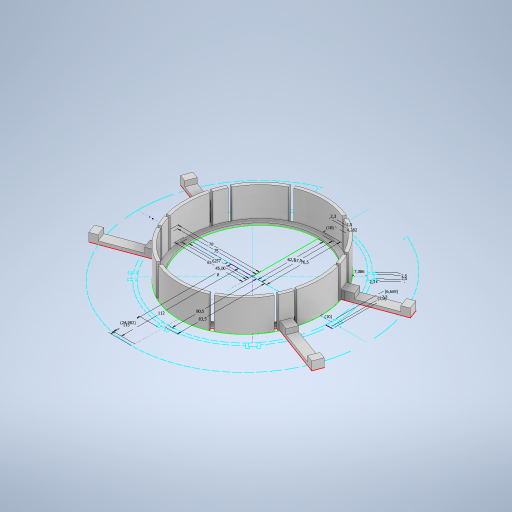
# Autodesk Inventor part: calibracao(0,5cm)
Saved by Autodesk Inventor 2024.3 (Build 283343000, 343)
## iProperties
Created: 2024-12-11
Part Number: calibracao(0,5cm)
Material: Genérico
Document SubType Name: Modeling
Designer: lostv
Density: 1 g/cm^3
Appearance: Padrão
Author: lostv
Autodesk Inventor part; units mm, degrees
ref_plane "YZ Plane" through (0, 0, 0) normal (1, 0, 0) x (0, 1, 0)
ref_plane "XZ Plane" through (0, 0, 0) normal (0, 1, 0) x (-1, 0, 0)
ref_plane "XY Plane" through (0, 0, 0) normal (0, 0, 1) x (1, 0, 0)
sketch "Esboço1" plane through (0, 0, 0) normal (0, 1, 0) x (-1, 0, 0)
  ellipse E0 centre (-16.8231, 43.9447) end of major axis (58.1769, 43.9447) minor radius 80.5 (58.1769, 43.9447) -> (-16.8231, 124.4447) ccw
  line L0 (-16.8231, 124.4447) -> (-16.8231, 43.9447) construction
  line L1 (-16.8231, 43.9447) -> (58.1769, 43.9447)
  line L2 (-16.8231, 43.9447) -> (38.0514, 98.8191) construction
  line L3 (-16.8231, 43.9447) -> (60.7811, 43.9447) construction
  line L4 (58.1769, 43.9447) -> (61.1769, 43.9447)
  ellipse E1 centre (-16.8231, 43.9447) end of major axis (-16.8231, 127.4447) minor radius 78 (36.942, 104.4388) -> (-11.8231, 127.273) ccw
  ellipse E2 centre (-16.8231, 43.9447) end of major axis (-16.8231, 127.4447) minor radius 78 (61.0369, 48.9447) -> (43.4965, 96.8842) ccw
  ellipse E3 centre (-16.8231, 43.9447) end of major axis (-16.8231, 127.4447) minor radius 78 (-21.8231, 127.273) -> (-70.5882, 104.4388) ccw
  ellipse E4 centre (-16.8231, 43.9447) end of major axis (-91.8231, 43.9447) minor radius 80.5 (-16.8231, 124.4447) -> (-91.8231, 43.9447) ccw
  line L5 (-16.8231, 43.9447) -> (-71.6976, 98.8191) construction
  line L6 (-16.8231, 43.9447) -> (-91.8231, 43.9447) construction
  line L7 (-16.8231, 43.9447) -> (-91.8231, 43.9447)
  ellipse E5 centre (-16.8231, 43.9447) end of major axis (-16.8231, 127.4447) minor radius 78 (-77.1427, 96.8842) -> (-94.6831, 48.9447) ccw
  line L8 (-96.047, 46.9447) -> (-91.771, 46.9447)
  line L9 (58.1769, 43.9447) -> (-91.8231, 43.9447)
  line L10 (-16.8231, 43.9447) -> (38.0514, -10.9298) construction
  ellipse E6 centre (-16.8231, 43.9447) end of major axis (58.1769, 43.9447) minor radius 80.5 (-16.8231, -36.5553) -> (58.1769, 43.9447) ccw
  line L11 (-16.8231, -36.5553) -> (-16.8231, 43.9447) construction
  line L12 (-13.8231, -40.7731) -> (-13.8231, -36.4909)
  line L13 (-11.8231, -40.7731) -> (-11.8231, -36.3762)
  line L14 (-13.8231, -36.4909) -> (-13.8231, -40.7731)
  ellipse E7 centre (-16.8231, 43.9447) end of major axis (-16.8231, -39.5553) minor radius 78 (-11.8231, -39.3836) -> (36.942, -16.5494) ccw
  ellipse E8 centre (-16.8231, 43.9447) end of major axis (-16.8231, -39.5553) minor radius 78 (43.4965, -8.9948) -> (61.0369, 38.9447) ccw
  line L15 (-69.7437, -13.0978) -> (-72.9021, -15.9416)
  line L16 (-73.673, -8.5619) -> (-76.9169, -11.4827)
  line L17 (-73.673, -8.5619) -> (-76.9169, -11.4827)
  line L18 (-69.7437, -13.0978) -> (-72.9021, -15.9416)
  line L19 (-19.8231, -40.7731) -> (-19.8231, -36.4909)
  line L20 (-19.8231, -36.4909) -> (-19.8231, -40.7731)
  line L21 (-21.8231, -40.7731) -> (-21.8231, -36.3762)
  ellipse E9 centre (-16.8231, 43.9447) end of major axis (-16.8231, -39.5553) minor radius 78 (-70.5882, -16.5494) -> (-21.8231, -39.3836) ccw
  line L22 (-16.8231, 43.9447) -> (-71.6976, -10.9298) construction
  ellipse E10 centre (-16.8231, 43.9447) end of major axis (-91.8231, 43.9447) minor radius 80.5 (-91.8231, 43.9447) -> (-16.8231, -36.5553) ccw
  ellipse E11 centre (-16.8231, 43.9447) end of major axis (-16.8231, -39.5553) minor radius 78 (-94.6831, 38.9447) -> (-77.1427, -8.9948) ccw
  line L23 (-96.047, 40.9447) -> (-91.8, 40.9447)
  line L24 (-56.8231, -78.0731) -> (-56.8231, -78.0731)
  line L25 (-96.047, 38.9447) -> (-91.6783, 38.9447)
  line L26 (-96.047, 48.9447) -> (-91.6783, 48.9447)
  line L27 (-96.047, 38.9447) -> (-98.347, 38.9447) construction
  line L28 (-98.347, 38.9447) -> (-98.347, 41.4447) construction
  line L29 (-98.347, 41.4447) -> (-96.047, 41.4447) construction
  line L30 (-96.047, 38.9447) -> (-98.347, 38.9447)
  line L31 (-98.347, 41.4447) -> (-98.347, 38.9447)
  line L32 (-98.347, 41.4447) -> (-96.047, 41.4447)
  line L33 (-96.047, 41.4447) -> (-96.047, 40.9447)
  line L34 (-96.047, 46.9447) -> (-96.047, 46.4447)
  line L35 (-98.347, 46.4447) -> (-96.047, 46.4447)
  line L36 (-98.347, 46.4447) -> (-98.347, 48.9447)
  line L37 (-98.347, 48.9447) -> (-96.047, 48.9447)
  line L38 (-96.047, 40.9447) -> (-96.047, 41.4447) construction
  line L39 (-96.047, 46.4447) -> (-96.047, 46.9447) construction
  line L40 (-96.047, 41.4447) -> (-96.047, 46.4447)
  line L41 (-72.9021, -15.9416) -> (-76.9169, -11.4827) construction
  line L42 (-78.2551, -9.9964) -> (-74.9072, -6.9819)
  line L43 (-71.5638, -17.4279) -> (-68.3579, -14.5413)
  line L44 (-71.5638, -17.4279) -> (-73.2731, -18.9669)
  line L45 (-73.2731, -18.9669) -> (-74.9459, -17.109)
  line L46 (-74.9459, -17.109) -> (-73.2367, -15.57)
  line L47 (-72.9021, -15.9416) -> (-73.2367, -15.57)
  line L48 (-76.9169, -11.4827) -> (-73.2367, -15.57)
  line L49 (-78.2551, -9.9964) -> (-79.9644, -11.5354)
  line L50 (-79.9644, -11.5354) -> (-78.2915, -13.3933)
  line L51 (-78.2915, -13.3933) -> (-76.5823, -11.8543)
  line L52 (-13.8231, -40.7731) -> (-19.8231, -40.7731) construction
  line L53 (-21.8231, -40.7731) -> (-21.8231, -43.0731)
  line L54 (-21.8231, -43.0731) -> (-19.3231, -43.0731)
  line L55 (-19.3231, -43.0731) -> (-19.3231, -40.7731)
  line L56 (-19.8231, -40.7731) -> (-19.3231, -40.7731)
  line L57 (-11.8231, -40.7731) -> (-11.8231, -43.0731)
  line L58 (-11.8231, -43.0731) -> (-14.3231, -43.0731)
  line L59 (-14.3231, -43.0731) -> (-14.3231, -40.7731)
  line L60 (-13.8231, -40.7731) -> (-14.3231, -40.7731)
  line L61 (-19.3231, -40.7731) -> (-14.3231, -40.7731)
  line L62 (46.3182, -11.5354) -> (44.6453, -13.3933)
  line L63 (44.6089, -9.9964) -> (46.3182, -11.5354)
  line L64 (44.6453, -13.3933) -> (42.9361, -11.8543)
  line L65 (40.0268, -8.5619) -> (43.2707, -11.4827)
  line L66 (44.6089, -9.9964) -> (41.261, -6.9819)
  line L67 (43.2707, -11.4827) -> (39.5905, -15.57)
  line L68 (39.2559, -15.9416) -> (43.2707, -11.4827) construction
  line L69 (36.0975, -13.0978) -> (39.2559, -15.9416)
  line L70 (39.2559, -15.9416) -> (39.5905, -15.57)
  line L71 (41.2997, -17.109) -> (39.5905, -15.57)
  line L72 (39.6269, -18.9669) -> (41.2997, -17.109)
  line L73 (37.9176, -17.4279) -> (39.6269, -18.9669)
  line L74 (37.9176, -17.4279) -> (34.7117, -14.5413)
  line L75 (62.4009, 38.9447) -> (64.7009, 38.9447)
  line L76 (64.7009, 38.9447) -> (64.7009, 41.4447)
  line L77 (64.7009, 41.4447) -> (62.4009, 41.4447)
  line L78 (62.4009, 41.4447) -> (62.4009, 40.9447)
  line L79 (62.4009, 40.9447) -> (58.1538, 40.9447)
  line L80 (62.4009, 38.9447) -> (58.0321, 38.9447)
  line L81 (62.4009, 41.4447) -> (62.4009, 46.4447)
  line L82 (64.7009, 46.4447) -> (62.4009, 46.4447)
  line L83 (62.4009, 46.9447) -> (62.4009, 46.4447)
  line L84 (64.7009, 46.4447) -> (64.7009, 48.9447)
  line L85 (64.7009, 48.9447) -> (62.4009, 48.9447)
  line L86 (62.4009, 48.9447) -> (58.0321, 48.9447)
  line L87 (62.4009, 46.9447) -> (58.1248, 46.9447)
  line L88 (39.2559, 103.831) -> (39.5905, 103.4594)
  line L89 (37.9176, 105.3172) -> (39.6269, 106.8562)
  line L90 (39.6269, 106.8562) -> (41.2997, 104.9984)
  line L91 (41.2997, 104.9984) -> (39.5905, 103.4594)
  line L92 (39.2559, 103.831) -> (43.2707, 99.3721) construction
  line L93 (43.2707, 99.3721) -> (39.5905, 103.4594)
  line L94 (44.6453, 101.2827) -> (42.9361, 99.7437)
  line L95 (46.3182, 99.4248) -> (44.6453, 101.2827)
  line L96 (44.6089, 97.8858) -> (46.3182, 99.4248)
  line L97 (44.6089, 97.8858) -> (41.261, 94.8713)
  line L98 (40.0268, 96.4513) -> (43.2707, 99.3721)
  line L99 (36.0975, 100.9871) -> (39.2559, 103.831)
  line L100 (37.9176, 105.3172) -> (34.7117, 102.4306)
  line L101 (-71.5638, 105.3172) -> (-68.3579, 102.4306)
  line L102 (-71.5638, 105.3172) -> (-73.2731, 106.8562)
  line L103 (-73.2731, 106.8562) -> (-74.9459, 104.9984)
  line L104 (-74.9459, 104.9984) -> (-73.2367, 103.4594)
  line L105 (-72.9021, 103.831) -> (-73.2367, 103.4594)
  line L106 (-69.7437, 100.9871) -> (-72.9021, 103.831)
  line L107 (-76.9169, 99.3721) -> (-73.2367, 103.4594)
  line L108 (-78.2915, 101.2827) -> (-76.5823, 99.7437)
  line L109 (-73.673, 96.4513) -> (-76.9169, 99.3721)
  line L110 (-79.9644, 99.4248) -> (-78.2915, 101.2827)
  line L111 (-78.2551, 97.8858) -> (-79.9644, 99.4248)
  line L112 (-78.2551, 97.8858) -> (-74.9072, 94.8713)
  line L113 (-21.8231, 128.6625) -> (-21.8231, 130.9625)
  line L114 (-21.8231, 128.6625) -> (-21.8231, 124.2656)
  line L115 (-21.8231, 130.9625) -> (-19.3231, 130.9625)
  line L116 (-19.3231, 130.9625) -> (-19.3231, 128.6625)
  line L117 (-19.8231, 128.6625) -> (-19.3231, 128.6625)
  line L118 (-19.8231, 128.6625) -> (-19.8231, 124.3803)
  line L119 (-19.3231, 128.6625) -> (-14.3231, 128.6625)
  line L120 (-14.3231, 130.9625) -> (-14.3231, 128.6625)
  line L121 (-11.8231, 130.9625) -> (-14.3231, 130.9625)
  line L122 (-11.8231, 128.6625) -> (-11.8231, 124.2656)
  line L123 (-11.8231, 128.6625) -> (-11.8231, 130.9625)
  line L124 (-13.8231, 128.6625) -> (-13.8231, 124.3803)
  line L125 (-13.8231, 128.6625) -> (-19.8231, 128.6625) construction
  line L126 (-13.8231, 128.6625) -> (-14.3231, 128.6625)
  line L127 (58.1538, 40.9447) -> (58.1248, 40.9447)
  line L128 (-91.8, 40.9447) -> (-91.771, 40.9447)
  line L129 (-16.8231, 43.9447) -> (-16.8231, 155.9447) construction
  line L130 (-16.8231, 43.9447) -> (89.6769, 43.9447) construction
  line L131 (-16.8231, 43.9447) -> (-16.8231, -64.5553) construction
  line L132 (-16.8231, 43.9447) -> (-123.3231, 43.9447) construction
  line L133 (-16.8231, 43.9447) -> (92.6769, 43.9447) construction
  line L134 (-16.8231, 43.9447) -> (-126.3231, 43.9447) construction
  line L135 (-16.8231, 43.9447) -> (-16.8231, 158.9447) construction
  line L136 (-16.8231, 43.9447) -> (-16.8231, -67.5553) construction
  line L137 (-14.3231, -43.0731) -> (-14.3231, -40.7731)
  line L138 (-19.3231, -40.7731) -> (-19.3231, -43.0731)
  line L139 (-19.3231, -40.7731) -> (-14.3231, -40.7731)
  ellipse E12 centre (-16.8231, 43.9447) end of major axis (92.6769, 43.9447) minor radius 115 (23.1769, -63.1078) -> (-56.8231, -63.1078) ccw
  line L140 (-123.2361, 93.6335) -> (-77.9442, 76.9085)
  line L141 (-80.7744, 68.1314) -> (-126.4279, 84.99)
  line L142 (-126.4279, 84.99) -> (-123.2361, 93.6335)
  line L143 (-16.8231, 43.9447) -> (-16.8231, -26.5553) construction
  line L144 (-16.8231, 43.9447) -> (48.1769, 43.9447) construction
  ellipse E13 centre (-16.8231, 43.9447) end of major axis (-16.8231, -26.5553) minor radius 65
  line L145 (-16.8231, 43.9447) -> (-16.8231, -23.5553) construction
  line L146 (-16.8231, 43.9447) -> (45.1769, 43.9447) construction
  ellipse E14 centre (-16.8231, 43.9447) end of major axis (-16.8231, -23.5553) minor radius 62
  line L147 (7.3874, 109.3718) -> (6.1319, 106.6478)
  line L148 (10.7346, 107.795) -> (9.4748, 105.0719)
  line L149 (7.3874, -21.4825) -> (6.1319, -18.7584)
  line L150 (10.7346, -19.9057) -> (9.4748, -17.1825)
  line L151 (-41.0336, 109.3718) -> (-39.7781, 106.6478)
  line L152 (-44.3808, 107.795) -> (-43.121, 105.0719)
  line L153 (-41.0336, -21.4825) -> (-39.7781, -18.7584)
  line L154 (-44.3808, -19.9057) -> (-43.121, -17.1825)
  line L155 (-73.0655, 79.2871) -> (-70.3521, 78.0032)
  line L156 (-71.612, 75.5393) -> (-74.3698, 76.7241)
  line L157 (-75.7143, 65.0508) -> (-78.6067, 65.8471)
  line L158 (-76.3169, 62.9424) -> (-79.201, 63.7668)
  line L159 (39.4193, 79.2871) -> (36.7059, 78.0032)
  line L160 (37.9658, 75.5393) -> (40.7236, 76.7241)
  line L161 (42.0681, 65.0508) -> (44.9605, 65.8471)
  line L162 (42.6707, 62.9424) -> (45.5548, 63.7668)
  line L163 (-73.0655, 8.6022) -> (-70.3521, 9.8862)
  line L164 (-71.612, 12.3501) -> (-74.3698, 11.1653)
  line L165 (-75.7143, 22.8386) -> (-78.6067, 22.0423)
  line L166 (-76.3169, 24.947) -> (-79.201, 24.1225)
  line L167 (42.6707, 24.947) -> (45.5548, 24.1225)
  line L168 (42.0681, 22.8386) -> (44.9605, 22.0423)
  line L169 (37.9658, 12.3501) -> (40.7236, 11.1653)
  line L170 (39.4193, 8.6022) -> (36.7059, 9.8862)
  line L171 (-16.8231, 43.9447) -> (40.1769, 43.9447)
  line L172 (-16.8231, 43.9447) -> (-16.8231, -18.5553)
  ellipse E15 centre (-16.8231, 43.9447) end of major axis (40.1769, 43.9447) minor radius 62.5
  line L173 (-81.8231, 43.9447) -> (-91.8231, 43.9447) construction
  line L174 (-71.6976, -10.9298) -> (-64.6113, -3.8435) construction
  line L175 (-16.8231, -36.5553) -> (-16.8231, -26.5553) construction
  line L176 (-80.7744, 68.1314) -> (-73.6902, 65.8471)
  line L177 (-73.6902, 65.8471) -> (-70.5922, 74.1936)
  line L178 (-70.5922, 74.1936) -> (-77.9442, 76.9085)
  line L179 (89.5899, 93.6335) -> (44.298, 76.9085)
  line L180 (47.1282, 68.1314) -> (92.7817, 84.99)
  line L181 (92.7817, 84.99) -> (89.5899, 93.6335)
  line L182 (47.1282, 68.1314) -> (40.044, 65.8471)
  line L183 (40.044, 65.8471) -> (36.946, 74.1936)
  line L184 (36.946, 74.1936) -> (44.298, 76.9085)
  line L185 (-123.2361, -5.7442) -> (-77.9442, 10.9809)
  line L186 (-80.7744, 19.758) -> (-126.4279, 2.8994)
  line L187 (-126.4279, 2.8994) -> (-123.2361, -5.7442)
  line L188 (-80.7744, 19.758) -> (-73.6902, 22.0423)
  line L189 (-73.6902, 22.0423) -> (-70.5922, 13.6958)
  line L190 (-70.5922, 13.6958) -> (-77.9442, 10.9809)
  line L191 (92.7817, 2.8994) -> (89.5899, -5.7442)
  line L192 (89.5899, -5.7442) -> (44.298, 10.9809)
  line L193 (47.1282, 19.758) -> (92.7817, 2.8994)
  line L194 (36.946, 13.6958) -> (44.298, 10.9809)
  line L195 (47.1282, 19.758) -> (40.044, 22.0423)
  line L196 (40.044, 22.0423) -> (36.946, 13.6958)
  point P0 (0, 0)
  point P1 (78.1769, 43.9447)
  point P2 (81.1769, 43.9447)
  point P3 (-100.7855, 43.9447)
  point P4 (-72.3567, -15.4505)
  point P5 (-97.197, 41.4447)
  point P6 (-97.197, 38.9447)
  point P7 (-96.047, 41.1947)
  point P8 (-96.047, 46.6947)
  point P9 (-97.197, 48.9447)
  point P10 (-93.8627, 48.9447)
  point P11 (-72.4185, -18.1974)
  point P12 (-77.4369, -12.6238)
  point P13 (-79.128, -12.4643)
  point P14 (-14.3231, -41.9231)
  point P15 (-19.5731, -40.7731)
  point P16 (-13.8231, -38.632)
  point P17 (62.4009, 41.1947)
  point P18 (-96.047, 43.9447)
  point P19 (-58.2564, -59.4853)
  point P20 (24.6102, -59.4853)
  point P21 (23.1769, -57.0582)
  point P22 (-13.0731, 130.9625)
  point P23 (64.7009, 40.1947)
  point P24 (-39.7781, -18.7584)
  point P25 (-41.0336, -21.4825)
  point P26 (7.3874, -21.4825)
  point P27 (6.1319, -18.7584)
  point P28 (-44.3808, -19.9057)
  point P29 (-43.121, -17.1825)
  point P30 (-43.121, 105.0719)
  point P31 (-44.3808, 107.795)
  point P32 (9.4748, -17.1825)
  point P33 (10.7346, -19.9057)
  point P34 (-41.0336, 109.3718)
  point P35 (-39.7781, 106.6478)
  point P36 (-82.3595, 68.7167)
  point P37 (-78.5767, 77.142)
  point P38 (-84.2338, 79.231)
  point P39 (-87.5779, 70.6437)
  point P40 (-119.9522, 82.5987)
  point P41 (-116.6506, 91.2017)
  point P42 (44.9605, 22.0423)
  point P43 (42.0681, 22.8386)
  point P44 (37.9658, 12.3501)
  point P45 (40.7236, 11.1653)
  point P46 (39.4193, 8.6022)
  point P47 (36.7059, 9.8862)
  point P48 (-70.3521, 9.8862)
  point P49 (-73.0655, 8.6022)
  point P50 (-74.3698, 11.1653)
  point P51 (-71.612, 12.3501)
  point P52 (-75.7143, 22.8386)
  point P53 (-78.6067, 22.0423)
  point P54 (-79.201, 24.1225)
  point P55 (-76.3169, 24.947)
  point P56 (45.5548, 63.7668)
  point P57 (42.6707, 62.9424)
  point P58 (42.6707, 24.947)
  point P59 (45.5548, 24.1225)
  point P60 (36.7059, 78.0032)
  point P61 (39.4193, 79.2871)
  point P62 (40.7236, 76.7241)
  point P63 (37.9658, 75.5393)
  point P64 (42.0681, 65.0508)
  point P65 (44.9605, 65.8471)
  point P66 (-78.1568, 67.2873)
  point P67 (-74.8288, 75.758)
  point P68 (-116.6506, -3.3123)
  point P69 (-119.9522, 5.2907)
  point P70 (-87.5779, 17.2456)
  point P71 (-84.2338, 8.6583)
  point P72 (-74.8288, 12.1313)
  point P73 (-78.1568, 20.602)
  point P74 (86.306, 5.2907)
  point P75 (83.0044, -3.3123)
  point P76 (50.5876, 8.6583)
  point P77 (53.9317, 17.2456)
  point P78 (44.5106, 20.602)
  point P79 (41.1826, 12.1313)
  point P80 (83.0044, 91.2017)
  point P81 (86.306, 82.5987)
  point P82 (44.5106, 67.2873)
  point P83 (53.9317, 70.6437)
  point P84 (50.5876, 79.231)
  point P85 (41.1826, 75.758)
  dimension "d3" = 83.5
  dimension "d4" = 78
  dimension "d0" = 75
  dimension "d1" = 80.5
  dimension "d2" = 45
  dimension "d7" = 2.3
  dimension "d8" = 2.3
  dimension "d11" = 6.6688
  dimension "d12" = 2.5
  dimension "d13" = 2.5
  dimension "d14" = 2.3
  dimension "d15" = 2.5
  dimension "d17" = 2.3
  dimension "d18" = 4.2822
  dimension "d20" = 112
  dimension "d25" = 115
  dimension "d26" = 24.9822
  dimension "d34" = 70.5
  dimension "d35" = 65
  dimension "d36" = 67.5
  dimension "d37" = 62
  dimension "d46" = 57
  dimension "d47" = 62.5
  dimension "d48" = 10
  dimension "d49" = 7.0863
  dimension "d50" = 10
  constraints: 394 end point, 149 symmetric about line, 51 point on line, 18 perpendicular, 16 coincident, 15 midpoint, 14 vertical, 13 collinear, 11 horizontal, 1 equal length, 118 other
  measures "d0" distance of L1.start L1.end
  measures "d1" distance of L0.start L1.start
  measures "d2" angle of L3 L2
  measures "d7" distance from line of point (-96.047, 41.195) L31
  measures "d8" distance from line of point (-96.047, 46.695) L36
  measures "d11" distance of L25.end L27.end
  measures "d12" distance from line of point (-72.418, -18.197) L46
  measures "d13" distance from line of point (-77.437, -12.624) L49
  measures "d14" distance between parallel lines of L41 L50
  measures "d15" distance between parallel lines of L55 L53
  measures "d17" distance from line of point (-19.573, -40.773) L54
  measures "d18" distance of L56.start L20.start
  measures "d20" distance of L130.start L129.end
  measures "d25" distance of L133.start L135.end
  measures "d26" vertical distance of point (-13.073, 130.962) L129.end
  measures "d34" distance of L143.start L143.end
  measures "d35" distance of L143.start L144.end
  measures "d36" distance of L145.start L145.end
  measures "d37" distance of L145.start L146.end
  measures "d46" distance of L171.start L171.end
  measures "d47" distance of L172.start L172.end
  measures "d48" distance of L173.start L9.end
  measures "d49" horizontal distance of L174.end L22.end
  measures "d50" distance of L11.start L143.end
extrude "Extrusão1" add sketch "Esboço1" along normal blind 2 contours E14 L195 L196 L194 L190 L189 L188 L7 E15 L1 | L1 E15 L7 E14 L176 L177 L178 L184 L183 L182 | E14 L194 L196 L195 | L182 L183 L184 E14 | E14 L178 L177 L176 | L188 L189 L190 E14
extrude "Extrusão2" add sketch "Esboço1" along normal blind 30 contours E13 L167 E14 L1 | L1 E14 L162 E13 | E13 L195 E14 L168 | L161 E14 L182 E13 | E13 L194 E14 L195 | L182 E14 L184 E13 | E13 L169 E14 L194 | L184 E14 L160 E13 | E14 L166 E13 L7 | L7 E13 L158 E14 | E13 L150 E14 L170 | L159 E14 L148 E13 | L157 E13 L176 E14 | E14 L188 E13 L165 | L176 E13 L178 E14 | E14 L190 E13 L188 | E13 L153 E14 L149 | L147 E14 L151 E13 | L178 E13 L156 E14 | E14 L164 E13 L190 | L152 E14 L155 E13 | E14 L154 E13 L163
extrude "Extrusão5" add sketch "Esboço1" along normal blind 8 contours L180 L182 E13 L184 L179 E0 | E6 L192 L194 E13 L195 L193 | E12 L179 L181 L180 | L193 L191 L192 E12 | E12 L141 L142 L140 | E12 L185 L187 L186 | L140 L178 E13 L176 L141 E4 | E13 L190 L185 E10 L186 L188
extrude "Extrusão6" add sketch "Esboço1" along normal blind 3 contours E0 L179 E2 L180 | L193 E8 L192 E6 | E2 L179 E12 L180 | L193 E12 L192 E8 | L140 E5 L141 E12 | L140 E4 L141 E5 | L186 E11 L185 E12 | L186 E10 L185 E11
